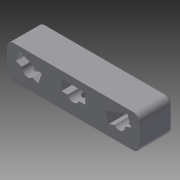
# Autodesk Inventor part: TSOP Cover
Saved by Autodesk Inventor 2015 (Build 190159000, 159)
## iProperties
Created: 2016-10-01
Part Number: TSOP Cover
Material: Generic
Document SubType Name: Modeling
Designer: James Yelland
Density: 1 g/cm^3
Appearance: Default
Author: James Yelland
Autodesk Inventor part; units mm, degrees
ref_plane "YZ Plane" through (0, 0, 0) normal (1, 0, 0) x (0, 1, 0)
ref_plane "XZ Plane" through (0, 0, 0) normal (0, 1, 0) x (-1, 0, 0)
ref_plane "XY Plane" through (0, 0, 0) normal (0, 0, 1) x (1, 0, 0)
sketch "Sketch1" plane through (0, 0, 0) normal (0, 1, 0) x (-1, 0, 0)
  line L0 (5.4, 3.85) -> (-5.4, 3.85)
  arc A0 (-2.5807, -0.95) -> (2.5807, -0.95) centre (0, 0) ccw
  line L1 (5.4, -0.95) -> (2.5807, -0.95)
  line L2 (5.4, -0.95) -> (5.4, 3.85)
  line L3 (-5.4, 3.85) -> (-5.4, -0.95)
  line L4 (-2.5807, -0.95) -> (-5.4, -0.95)
  line L5 (14.2866, 1.2915) -> (15.9283, -3.2191)
  line L6 (18.5775, -2.2548) -> (15.9283, -3.2191)
  arc A1 (18.5775, -2.2548) -> (23.4277, -0.4895) centre (20.6777, -0.4794) ccw
  line L7 (24.4352, 4.9853) -> (14.2866, 1.2915)
  line L8 (26.0769, 0.4748) -> (24.4352, 4.9853)
  line L9 (26.0769, 0.4748) -> (23.4277, -0.4895)
  line L10 (-24.4352, 4.9853) -> (-26.0769, 0.4748)
  line L11 (-23.4277, -0.4895) -> (-26.0769, 0.4748)
  arc A2 (-23.4277, -0.4895) -> (-18.5775, -2.2548) centre (-20.6777, -0.4794) ccw
  line L12 (-14.2866, 1.2915) -> (-24.4352, 4.9853)
  line L13 (-15.9283, -3.2191) -> (-14.2866, 1.2915)
  line L14 (-15.9283, -3.2191) -> (-18.5775, -2.2548)
  line L15 (-30, 4.0495) -> (-30, -4.9505)
  line L16 (30, 4.0495) -> (30, -4.9505)
  line L17 (-27, -7.9505) -> (27, -7.9505)
  line L18 (27, 7.0495) -> (-27, 7.0495)
  arc A3 (-30, -4.9505) -> (-27, -7.9505) centre (-27, -4.9505) ccw
  arc A4 (27, -7.9505) -> (30, -4.9505) centre (27, -4.9505) ccw
  arc A5 (30, 4.0495) -> (27, 7.0495) centre (27, 4.0495) ccw
  arc A6 (-27, 7.0495) -> (-30, 4.0495) centre (-27, 4.0495) ccw
  point P0 (0, 0)
  point P1 (30, 7.0495)
  point P2 (-30, 7.0495)
  dimension "d2" = 60
  dimension "d42" = 3
  constraints: 38 end point, 14 point on circle, 8 tangent, 7 centre point, 4 point on line, 3 equal radius, 2 vertical, 1 horizontal, 1 parallel
  measures "d2" distance of point (30, 7.05) point (-30, 7.05)
  measures "d42" radius of A3
extrude "Extrusion1" add sketch "Sketch1" along normal blind 15
sketch "Sketch2" plane through (0, 15, 0) normal (0, 1, 0) x (1, 0, 0)
  line L0 (24.4352, -4.9853) -> (14.2866, -1.2915) projected
  line L1 (14.2866, -1.2915) -> (15.9283, 3.2191) projected
  line L2 (15.9283, 3.2191) -> (18.5775, 2.2548) projected
  arc A0 (23.4277, 0.4895) -> (18.5775, 2.2548) centre (20.6777, 0.4794) ccw projected
  line L3 (23.4277, 0.4895) -> (26.0769, -0.4748) projected
  line L4 (26.0769, -0.4748) -> (24.4352, -4.9853) projected
  line L5 (-14.2866, -1.2915) -> (-24.4352, -4.9853) projected
  line L6 (-24.4352, -4.9853) -> (-26.0769, -0.4748) projected
  line L7 (-26.0769, -0.4748) -> (-23.4277, 0.4895) projected
  arc A1 (-18.5775, 2.2548) -> (-23.4277, 0.4895) centre (-20.6777, 0.4794) ccw projected
  line L8 (-18.5775, 2.2548) -> (-15.9283, 3.2191) projected
  line L9 (-15.9283, 3.2191) -> (-14.2866, -1.2915) projected
  line L10 (-5.4, -3.85) -> (-5.4, 0.95) projected
  line L11 (-5.4, 0.95) -> (-2.5807, 0.95) projected
  arc A2 (2.5807, 0.95) -> (-2.5807, 0.95) centre (0, 0) ccw projected
  line L12 (2.5807, 0.95) -> (5.4, 0.95) projected
  line L13 (5.4, 0.95) -> (5.4, -3.85) projected
  line L14 (5.4, -3.85) -> (-5.4, -3.85) projected
  line L15 (27, 7.9505) -> (-27, 7.9505) projected
  arc A3 (-27, 7.9505) -> (-30, 4.9505) centre (-27, 4.9505) ccw projected
  line L16 (-30, 4.9505) -> (-30, -4.0495) projected
  arc A4 (-30, -4.0495) -> (-27, -7.0495) centre (-27, -4.0495) ccw projected
  line L17 (-27, -7.0495) -> (27, -7.0495) projected
  arc A5 (27, -7.0495) -> (30, -4.0495) centre (27, -4.0495) ccw projected
  line L18 (30, -4.0495) -> (30, 4.9505) projected
  arc A6 (30, 4.9505) -> (27, 7.9505) centre (27, 4.9505) ccw projected
extrude "Extrusion2" add sketch "Sketch2" against normal blind 2 contours L0 L1 L2 A0 L3 L4 | L5 L6 L7 A1 L8 L9 | L10 L11 A2 L12 L13 L14 | A6 L18 A5 L17 A4 L16 A3 L15
sketch "Sketch3" plane through (-14.2866, 0, 1.2915) normal (-0.3420201, 0, -0.9396926) x (-0.9396926, 0, 0.3420201)
  line L0 (10.8, 0) -> (0, 0) projected
  line L1 (5.4, 0) -> (18.9092, 0) construction
  line L2 (5.4, 0) -> (5.4, 9.5)
  arc A0 (6.9, 9.5) -> (3.9, 9.5) centre (5.4, 9.5) ccw
  line L3 (3.9, 9.5) -> (3.9, 5.5)
  line L4 (6.9, 9.5) -> (6.9, 5.5)
  arc A1 (3.9, 5.5) -> (6.9, 5.5) centre (5.4, 5.5) ccw
  point P0 (-13.8667, 0)
  dimension "d10" = 9.5
  dimension "d18" = 1.5
  dimension "d19" = 4
  dimension "d20" = 4
  constraints: 8 end point, 4 point on circle, 3 vertical, 2 centre point, 1 coincident, 1 horizontal, 1 midpoint, 1 point on line
  measures "d10" distance of L1.start L2.end
  measures "d18" radius of A0
  measures "d19" distance of L3.start L3.end
  measures "d20" distance of L4.start L4.end
extrude "Extrusion3" cut sketch "Sketch3" along normal through all
sketch "Sketch4" plane through (5.4, 0, 3.85) normal (0, 0, -1) x (-1, 0, 0)
  line L0 (10.8, 0) -> (0, 0)
  line L1 (5.4, 0) -> (18.9092, 0) construction
  line L2 (5.4, 0) -> (5.4, 9.5)
  arc A0 (6.9, 9.5) -> (3.9, 9.5) centre (5.4, 9.5) ccw
  line L3 (3.9, 9.5) -> (3.9, 5.5)
  line L4 (6.9, 9.5) -> (6.9, 5.5)
  arc A1 (3.9, 5.5) -> (6.9, 5.5) centre (5.4, 5.5) ccw
  point P0 (5.4, 0)
  point P1 (-13.8667, 0)
  dimension "d23" = 9.5
  dimension "d24" = 1.5
  dimension "d25" = 4
  dimension "d26" = 4
  constraints: 10 end point, 4 point on circle, 3 vertical, 2 centre point, 1 coincident, 1 horizontal, 1 midpoint, 1 point on line
  measures "d23" distance of L1.start L2.end
  measures "d24" radius of A0
  measures "d25" distance of L3.start L3.end
  measures "d26" distance of L4.start L4.end
extrude "Extrusion4" cut sketch "Sketch4" along normal through all
sketch "Sketch5" plane through (24.4352, 0, 4.9853) normal (0.3420201, 0, -0.9396926) x (-0.9396926, 0, -0.3420201)
  line L0 (10.8, 0) -> (0, 0)
  line L1 (5.4, 0) -> (18.9092, 0) construction
  line L2 (5.4, 0) -> (5.4, 9.5)
  arc A0 (6.9, 9.5) -> (3.9, 9.5) centre (5.4, 9.5) ccw
  line L3 (3.9, 9.5) -> (3.9, 5.5)
  line L4 (6.9, 9.5) -> (6.9, 5.5)
  arc A1 (3.9, 5.5) -> (6.9, 5.5) centre (5.4, 5.5) ccw
  point P0 (24.6667, 0)
  point P1 (-13.8667, 0)
  dimension "d29" = 9.5
  dimension "d30" = 1.5
  dimension "d31" = 4
  dimension "d32" = 4
  constraints: 10 end point, 4 point on circle, 3 vertical, 2 centre point, 1 coincident, 1 horizontal, 1 midpoint, 1 point on line
  measures "d29" distance of L1.start L2.end
  measures "d30" radius of A0
  measures "d31" distance of L3.start L3.end
  measures "d32" distance of L4.start L4.end
extrude "Extrusion5" cut sketch "Sketch5" along normal through all
sketch "Sketch7" plane through (27, 0, -7.9505) normal (0, 0, -1) x (-1, 0, 0)
  line L0 (5.1994, 9.5) -> (5.1994, 5.5) projected
  ellipse E0 centre (3.6031, 5.5) end of major axis (2.0068, 5.5) minor radius 1.5 (2.0068, 5.5) -> (5.1994, 5.5) ccw projected
  line L1 (2.0068, 5.5) -> (2.0068, 9.5) projected
  ellipse E1 centre (3.6031, 9.5) end of major axis (5.1994, 9.5) minor radius 1.5 (5.1994, 9.5) -> (2.0068, 9.5) ccw projected
  line L2 (28.5, 9.5) -> (28.5, 5.5) projected
  arc A0 (25.5, 5.5) -> (28.5, 5.5) centre (27, 5.5) ccw projected
  line L3 (25.5, 5.5) -> (25.5, 9.5) projected
  arc A1 (28.5, 9.5) -> (25.5, 9.5) centre (27, 9.5) ccw projected
  line L4 (51.9932, 9.5) -> (51.9932, 5.5) projected
  ellipse E2 centre (50.3969, 5.5) end of major axis (48.8006, 5.5) minor radius 1.5 (48.8006, 5.5) -> (51.9932, 5.5) ccw projected
  line L5 (48.8006, 5.5) -> (48.8006, 9.5) projected
  ellipse E3 centre (50.3969, 9.5) end of major axis (51.9932, 9.5) minor radius 1.5 (51.9932, 9.5) -> (48.8006, 9.5) ccw projected
  line L6 (0, 0) -> (54, 0) projected
  arc A2 (30, 9.5) -> (24, 9.5) centre (27, 9.5) ccw
  arc A3 (24, 5.5) -> (30, 5.5) centre (27, 5.5) ccw
  line L7 (24, 9.5) -> (24, 5.5)
  line L8 (30, 5.5) -> (30, 9.5)
  line L9 (29.5807, 0) -> (29.5807, 15) projected
  line L10 (0, 0) -> (0, 15) projected
  line L11 (54, 0) -> (54, 15) projected
  line L12 (0, 15) -> (54, 15) projected
  point P0 (27, 0)
  point P1 (29.5807, 13)
  dimension "d43" = 3
  dimension "d44" = 3
  constraints: 4 end point, 4 point on circle, 2 centre point, 2 coincident, 1 parallel, 1 vertical, 4 other
  measures "d43" radius of A2
  measures "d44" radius of A3
extrude "Extrusion7" add sketch "Sketch7" along normal blind 2 contours L9 A2 L8 A3 | A3 L7 A2 L9
ref_plane "Work Plane1" through (-21.8006, 7.5, -7.9505) normal (-0.3420201, 0, -0.9396926) x (-0.9396926, 0, 0.3420201)
sketch "Sketch8" plane through (-21.8006, 7.5, -7.9505) normal (-0.3420201, 0, -0.9396926) x (-0.9396926, 0, 0.3420201)
  spline S0 degree 2 poles (0, -2) (0, -3.5) (1.5, -3.5) (3, -3.5) (3, -2) knots 0 0 0 0.5 0.5 1 1 1 weights 1 0.707107 1 0.707107 1 projected
  line L0 (3, -2) -> (3, 2) projected
  spline S1 degree 2 poles (3, 2) (3, 3.5) (1.5, 3.5) (0, 3.5) (0, 2) knots 0 0 0 0.5 0.5 1 1 1 weights 1 0.707107 1 0.707107 1 projected
  line L1 (0, 2) -> (0, -2) projected
  line L2 (3, -2) -> (1.5, -2)
  arc A0 (-1.5, -2) -> (4.5, -2) centre (1.5, -2) ccw
  arc A1 (4.5, 2) -> (-1.5, 2) centre (1.5, 2) ccw
  line L3 (4.5, -2) -> (4.5, 2)
  line L4 (-1.5, 2) -> (-1.5, -2)
  point P0 (-17.7667, -7.5)
  dimension "d50" = 1.5
  dimension "d51" = 3
  constraints: 6 end point, 4 point on circle, 2 centre point, 2 horizontal alignment, 1 coincident, 1 parallel, 1 perpendicular, 1 point on line, 1 vertical
  measures "d50" distance of L0.start L2.end
  measures "d51" radius of A0
extrude "Extrusion8" add sketch "Sketch8" along normal blind 2 and the other way blind 1
ref_plane "Work Plane2" through (21.8006, 7.5, -7.9505) normal (0.3420201, 0, -0.9396926) x (-0.9396926, 0, -0.3420201)
sketch "Sketch9" plane through (21.8006, 7.5, -7.9505) normal (0.3420201, 0, -0.9396926) x (-0.9396926, 0, -0.3420201)
  line L0 (-3, 2) -> (-3, -2) projected
  spline S0 degree 2 poles (-3, -2) (-3, -3.5) (-1.5, -3.5) (0, -3.5) (0, -2) knots 0 0 0 0.5 0.5 1 1 1 weights 1 0.707107 1 0.707107 1 projected
  line L1 (0, -2) -> (0, 2) projected
  spline S1 degree 2 poles (0, 2) (0, 3.5) (-1.5, 3.5) (-3, 3.5) (-3, 2) knots 0 0 0 0.5 0.5 1 1 1 weights 1 0.707107 1 0.707107 1 projected
  arc A0 (-4.5, -2) -> (1.5, -2) centre (-1.5, -2) ccw
  line L2 (1.5, -2) -> (1.5, 2)
  line L3 (-4.5, -2) -> (-4.5, 2)
  arc A1 (1.5, 2) -> (-4.5, 2) centre (-1.5, 2) ccw
  point P0 (17.7667, -7.5)
  dimension "d56" = 3
  dimension "d57" = 4
  constraints: 4 end point, 4 point on circle, 2 centre point, 2 horizontal alignment, 2 vertical
  measures "d56" radius of A0
  measures "d57" distance of L2.start L2.end
extrude "Extrusion9" add sketch "Sketch9" along normal blind 2 and the other way blind 1
chamfer "Chamfer3" distance 0.35 angle 45 12 edges at (-21.0751, 7.5, -10.3429) (-23.8942, 2.5, -9.3168) (-26.7133, 7.5, -8.2908) (-23.8942, 12.5, -9.3168) (0, 12.5, -9.9505) (3, 7.5, -9.9505) (0, 2.5, -9.9505) (-3, 7.5, -9.9505) (23.8942, 12.5, -9.3168) (26.7133, 7.5, -8.2908) (23.8942, 2.5, -9.3168) (21.0751, 7.5, -10.3429)
chamfer "Chamfer4" distance 1 angle 45 8 edges at (0, 15, -7.9505) (-29.1213, 15, -7.0718) (-30, 15, -0.4505) (-29.1213, 15, 6.1709) (0, 15, 7.0495) (29.1213, 15, 6.1709) (30, 15, -0.4505) (29.1213, 15, -7.0718)
body "Solid1"
